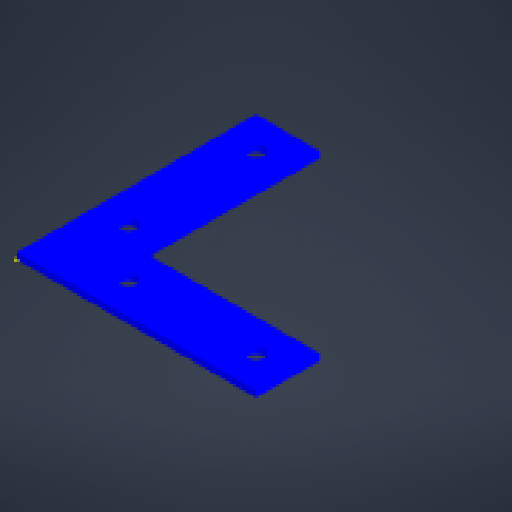
# Autodesk Inventor part: Деталь3
Saved by Autodesk Inventor 2024 (Build 280153000, 153)
## iProperties
Created: 2023-09-25
Part Number: Деталь3
Material: Типовые
Document SubType Name: Modeling
Designer: user
Density: 1 g/cm^3
Appearance: По умолчанию
Author: user
Autodesk Inventor part; units mm, degrees
ref_plane "YZ Plane" through (0, 0, 0) normal (1, 0, 0) x (0, 1, 0)
ref_plane "XZ Plane" through (0, 0, 0) normal (0, 1, 0) x (-1, 0, 0)
ref_plane "XY Plane" through (0, 0, 0) normal (0, 0, 1) x (1, 0, 0)
sketch "Эскиз1" plane through (0, 0, 0) normal (0, 0, 1) x (1, 0, 0)
  line L0 (0, 0) -> (75, 0)
  line L1 (20, 20) -> (20, 75)
  line L2 (0, 75) -> (0, 0)
  line L3 (20, 20) -> (75, 20)
  circle A0 centre (10, 131.9318) radius 2.5
  circle A1 centre (10, 65) radius 2.5
  circle A2 centre (10, 25) radius 2.5
  circle A3 centre (25, 10) radius 2.5
  circle A4 centre (65, 10) radius 2.5
  line L4 (0, 75) -> (20, 75)
  line L5 (75, 0) -> (75, 20)
  point P0 (10, 75)
  point P1 (75, 10)
  dimension "d5" = 5
  dimension "d11" = 20
  dimension "d12" = 20
  dimension "d13" = 75
  dimension "d14" = 10
  dimension "d15" = 40
  dimension "d16" = 10
  dimension "d17" = 40
  constraints: 12 end point, 5 centre point, 4 equal radius, 4 perpendicular, 3 vertical alignment, 2 horizontal, 2 horizontal alignment, 2 midpoint, 1 parallel
  measures "d5" diameter of A0
  measures "d11" distance of L0.end L3.end
  measures "d12" distance of L2.start L1.end
  measures "d13" distance of L0.start L0.end
  measures "d14" horizontal distance of L2.start A1.centre
  measures "d15" distance of A1.centre A2.centre
  measures "d16" horizontal distance of A4.centre L0.end
  measures "d17" distance of A3.centre A4.centre
extrude "Выдавливание1" add sketch "Эскиз1" against normal blind 2 contours L2 L4 L1 L3 L5 L0
sketch "Эскиз2" plane through (0, 0, -2) normal (0, 0, -1) x (-1, 0, 0)
  circle A0 centre (-6.5, 6.5) radius 2.25
  circle A1 centre (-48.5, 6.5) radius 2.25
  point P0 (0, 0)
  dimension "d20" = 6.5
  dimension "d21" = 6.5
  dimension "d22" = 4.5
  dimension "d23" = 42
  constraints: 2 centre point, 1 equal radius, 1 horizontal alignment
  measures "d20" horizontal distance of point (0, 0) A0.centre
  measures "d21" horizontal distance of point (0, 0) A0.centre
  measures "d22" diameter of A0
  measures "d23" distance of A1.centre A0.centre
extrude "Выдавливание2" cut sketch "Эскиз2" against normal through all
equation "\"d16\" = d14"
equation "\"d17\" = d15"
